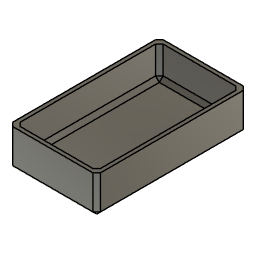
Bucket v4 (Autodesk Fusion 360 design; units mm, degrees)
Autodesk Fusion 360 part; units mm, degrees
sketch "Sketch1" plane through (0, 0, 0) normal (0, 0, 1) x (1, 0, 0)
  line L0 (35, 60) -> (-35, 60)
  line L1 (-35, 60) -> (-35, -60)
  line L2 (-35, -60) -> (35, -60)
  line L3 (35, -60) -> (35, 60)
  line L4 (35, 60) -> (-35, -60) construction
  line L5 (-35, 60) -> (35, -60) construction
  dimension "d1" = 70
  dimension "d2" = 120
  constraint horizontal L0
  constraint perpendicular L0 L1
  constraint parallel L0 L2
  constraint parallel L1 L3
  constraint coincident L4 origin
  constraint coincident L5 origin
  measures "d1" distance of L1.end L2.end
  measures "d2" distance of L0.end L1.end
extrude "Extrude1" add sketch "Sketch1" along normal blind 5
sketch "Sketch2" plane through (0, 0, 5) normal (0, 0, 1) x (-1, 0, 0)
  line L0 (-35, 60) -> (-35, -60)
  line L1 (-35, -60) -> (35, -60)
  line L2 (35, -60) -> (35, 60)
  line L3 (35, 60) -> (-35, 60)
  line L4 (32, 57) -> (-32, 57)
  line L5 (-32, 57) -> (-32, -57)
  line L6 (-32, -57) -> (32, -57)
  line L7 (32, -57) -> (32, 57)
  dimension "d5" = -3
extrude "Extrude2" add sketch "Sketch2" along normal blind 25
chamfer "Chamfer1" distance 3 angle 45 12 edges at (35, -60, 15) (-35, -60, 15) (35, 60, 15) (-35, 60, 15) (-32, 57, 17.5) (0, 57, 5) (-32, 0, 5) (32, 57, 17.5) (32, 0, 5) (32, -57, 17.5) (0, -57, 5) (-32, -57, 17.5) 1 faces at (-11.6667, -20, 0)
